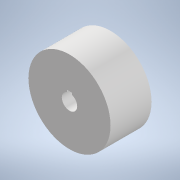
# Autodesk Inventor part: raHandController
Saved by Autodesk Inventor 2020.3 (Build 243373000, 373)
## iProperties
Created: 2020-05-28
Part Number: raHandController
Material: Generic
Document SubType Name: Modeling
Designer: robst
Density: 1 g/cm^3
Appearance: Default
Author: robst
Autodesk Inventor part; units mm, degrees
ref_plane "YZ Plane" through (0, 0, 0) normal (1, 0, 0) x (0, 1, 0)
ref_plane "XZ Plane" through (0, 0, 0) normal (0, 1, 0) x (-1, 0, 0)
ref_plane "XY Plane" through (0, 0, 0) normal (0, 0, 1) x (1, 0, 0)
sketch "Sketch1" plane through (0, 0, 0) normal (0, 0, 1) x (1, 0, 0)
  line L0 (-1.5939, 3.4346) -> (-1.5939, 4.6252) projected
  arc A0 (-1.5939, 4.6252) -> (1.5939, 4.6252) centre (0, 0.1373) ccw projected
  line L1 (1.5939, 4.6252) -> (1.5939, 3.4346) projected
  line L2 (1.5939, 3.4346) -> (-1.5939, 3.4346) projected
  arc A1 (-1.5939, 4.6252) -> (1.5939, 4.6252) centre (0, 0.1373) ccw
  line L3 (-1.5939, 4.6252) -> (-1.5939, 3.4346)
  line L4 (-1.5939, 3.4346) -> (1.5939, 3.4346)
  line L5 (1.5939, 3.4346) -> (1.5939, 4.6252)
  line L6 (-1.5939, 4.6252) -> (-1.5939, 5.8158)
  line L7 (-1.5939, 5.8158) -> (1.5939, 5.8158)
  line L8 (1.5939, 5.8158) -> (1.5939, 4.6252)
  circle A2 centre (0, 0.1373) radius 25.4
  point P0 (0, 0)
  dimension "d0" = 50.8
  constraints: 12 end point, 3 collinear, 2 centre point, 2 coincident, 2 point on circle, 2 vertical, 1 concentric, 1 horizontal, 1 perpendicular
  measures "d0" diameter of A2
extrude "Extrusion1" add sketch "Sketch1" against normal blind 25.4
body "Solid1"
